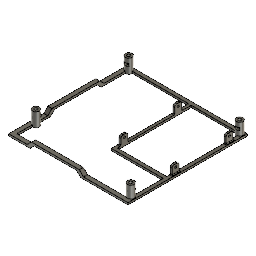
Mobo+HDD (Autodesk Fusion 360 design; units mm, degrees)
Autodesk Fusion 360 part; units mm, degrees
note: some values were not read from the file. Set by a fixed rule: which sketch regions a step uses.
sketch "Sketch4" plane through (0, 0, 0) normal (0, 0, 1) x (1, 0, 0)
  line L0 (0, 0) -> (170, 0)
  line L1 (170, 0) -> (170, 170)
  line L2 (170, 170) -> (0, 170)
  line L3 (0, 170) -> (0, 0)
  line L4 (165, 6) -> (165, 165)
  line L5 (165, 165) -> (6, 165)
  line L6 (6, 165) -> (6, 6)
  line L7 (6, 6) -> (165, 6)
  circle A0 centre (6, 33) radius 2.25
  circle A1 centre (6, 33) radius 5
  circle A2 centre (6, 165) radius 2.25
  circle A3 centre (6, 165) radius 5
  circle A4 centre (164, 10) radius 2.25
  circle A5 centre (164, 10) radius 5
  line L8 (165, 165) -> (95, 165)
  line L9 (95, 165) -> (95, 60)
  line L10 (95, 60) -> (165, 60)
  line L11 (165, 60) -> (165, 165)
  line L12 (91, 165) -> (91, 55)
  line L13 (91, 55) -> (165, 55)
  line L14 (0, 50) -> (6, 50)
  line L15 (0, 60) -> (6, 60)
  line L16 (0, 120) -> (6, 120)
  line L17 (0, 130) -> (6, 130)
  line L18 (26.6543, 6) -> (26.6543, 0)
  line L19 (36.6543, 6) -> (36.6543, 0)
  line L20 (96.6543, 6) -> (96.6543, 0)
  line L21 (106.6543, 6) -> (106.6543, 0)
  line L22 (92, 75) -> (95, 75)
  line L23 (95, 75) -> (95, 65)
  line L24 (95, 65) -> (92, 65)
  line L25 (92, 65) -> (92, 75)
  line L26 (165, 65) -> (168, 65)
  line L27 (168, 65) -> (168, 75)
  line L28 (168, 75) -> (165, 75)
  line L29 (165, 75) -> (165, 65)
  line L30 (95, 151.5) -> (92, 151.5)
  line L31 (92, 151.5) -> (92, 141.5)
  line L32 (92, 141.5) -> (95, 141.5)
  line L33 (95, 141.5) -> (95, 151.5)
  line L34 (165, 151.5) -> (168, 151.5)
  line L35 (168, 151.5) -> (168, 141.5)
  line L36 (168, 141.5) -> (165, 141.5)
  line L37 (165, 141.5) -> (165, 151.5)
  circle A6 centre (164, 165) radius 2.25
  circle A7 centre (164, 165) radius 5
  line L38 (6, 165) -> (6, 170) construction
  line L39 (6, 167.5) -> (170, 167.5) construction
  line L40 (165, 165) -> (170, 165) construction
  line L41 (167.5, 165) -> (167.5, 0) construction
  line L42 (6, 6) -> (0, 6) construction
  line L43 (3, 6) -> (3, 170) construction
  circle A8 centre (147, 167.5) radius 1.75
  circle A9 centre (157, 167.5) radius 1.75
  line L44 (147, 169.25) -> (157, 169.25)
  line L45 (157, 165.75) -> (147, 165.75)
  line L46 (0, 85) -> (170, 85) construction
  circle A10 centre (10.9777, 3) radius 1.75
  line L47 (10.9777, 4.75) -> (20.9777, 4.75)
  circle A11 centre (20.9777, 3) radius 1.75
  line L48 (10.9777, 1.25) -> (20.9777, 1.25)
  circle A12 centre (147, 2.5) radius 1.75
  circle A13 centre (157, 2.5) radius 1.75
  line L49 (147, 0.75) -> (157, 0.75)
  line L50 (157, 4.25) -> (147, 4.25)
  line L51 (0, 0) -> (39.1523, 39.1523) construction
  line L52 (0, 0) -> (55.3697, 0) construction
  line L53 (4.75, 10.9777) -> (4.75, 20.9777)
  circle A14 centre (3, 10.9777) radius 1.75
  line L54 (1.25, 10.9777) -> (1.25, 20.9777)
  circle A15 centre (3, 20.9777) radius 1.75
  line L55 (167.5, 12.0207) -> (164, 14.0415)
  line L56 (164, 14.0415) -> (160.5, 12.0207)
  line L57 (160.5, 12.0207) -> (160.5, 7.9793)
  line L58 (160.5, 7.9793) -> (164, 5.9585)
  line L59 (164, 5.9585) -> (167.5, 7.9793)
  line L60 (167.5, 7.9793) -> (167.5, 12.0207)
  line L61 (9.5, 35.0207) -> (6, 37.0415)
  line L62 (6, 37.0415) -> (2.5, 35.0207)
  line L63 (2.5, 35.0207) -> (2.5, 30.9793)
  line L64 (2.5, 30.9793) -> (6, 28.9585)
  line L65 (6, 28.9585) -> (9.5, 30.9793)
  line L66 (9.5, 30.9793) -> (9.5, 35.0207)
  line L67 (9.5, 167.0207) -> (6, 169.0415)
  line L68 (6, 169.0415) -> (2.5, 167.0207)
  line L69 (2.5, 167.0207) -> (2.5, 162.9793)
  line L70 (2.5, 162.9793) -> (6, 160.9585)
  line L71 (6, 160.9585) -> (9.5, 162.9793)
  line L72 (9.5, 162.9793) -> (9.5, 167.0207)
  line L73 (167.5, 167.0207) -> (164, 169.0415)
  line L74 (164, 169.0415) -> (160.5, 167.0207)
  line L75 (160.5, 167.0207) -> (160.5, 162.9793)
  line L76 (160.5, 162.9793) -> (164, 160.9585)
  line L77 (164, 160.9585) -> (167.5, 162.9793)
  line L78 (167.5, 162.9793) -> (167.5, 167.0207)
  line L79 (160.5, 162.9793) -> (160.5, 161.4293)
  line L80 (167.5, 162.9793) -> (167.5, 161.4293)
  line L81 (167.5, 12.0207) -> (167.5, 13.5707)
  line L82 (160.5, 12.0207) -> (160.5, 13.5707)
  line L83 (9.5, 35.0207) -> (9.5, 36.5707)
  line L84 (2.5, 35.0207) -> (2.5, 36.5707)
  line L85 (2.5, 162.9793) -> (2.5, 161.4293)
  line L86 (9.5, 162.9793) -> (9.5, 161.4293)
  line L87 (1.25, 145.7335) -> (1.25, 155.7335)
  circle A16 centre (3, 155.7335) radius 1.75
  line L88 (4.75, 145.7335) -> (4.75, 155.7335)
  circle A17 centre (3, 145.7335) radius 1.75
  point P0 (6, 33)
  point P1 (164, 10)
  point P2 (164, 165)
  point P3 (164, 10)
  point P4 (6, 33)
  point P5 (6, 165)
  point P6 (164, 165)
  dimension "d44" = 170
  dimension "d45" = 170
  dimension "d47" = 33
  dimension "d48" = 10
  dimension "d49" = 4.5
  dimension "d50" = 10
  dimension "d51" = 4.5
  dimension "d52" = 10
  dimension "d55" = 4.5
  dimension "d56" = 10
  dimension "d57" = 70
  dimension "d58" = 105
  dimension "d60" = 60
  dimension "d61" = 10
  dimension "d63" = 10
  dimension "d64" = 10
  dimension "d65" = 10
  dimension "d66" = 60
  dimension "d67" = 105
  dimension "d75" = 5
  dimension "d76" = 6
  dimension "d77" = 6
  dimension "d78" = 5
  dimension "d79" = 6
  dimension "d80" = 4
  dimension "d81" = 3
  dimension "d82" = 10
  dimension "d83" = 10
  dimension "d84" = 3
  dimension "d85" = 10
  dimension "d86" = 3
  dimension "d87" = 3
  dimension "d88" = 10
  dimension "d89" = 13.5
  dimension "d90" = 13.5
  dimension "d91" = 66.5
  dimension "d92" = 66.5
  dimension "d93" = 6
  dimension "d94" = 4.5
  dimension "d95" = 10
  dimension "d112" = 3.5
  dimension "d113" = 3.5
  dimension "d114" = 10
  dimension "d115" = 8
  dimension "d116" = 45
  dimension "d117" = 10
  dimension "d118" = 3.5
  dimension "d119" = 3.5
  dimension "d121" = 3.5
  dimension "d122" = 3.5
  dimension "d123" = 3.5
  dimension "d124" = 3.5
  dimension "d133" = 10
  dimension "d134" = 3.5
  dimension "d135" = 3.5
  constraint horizontal L0
  constraint vertical L1
  constraint horizontal L2
  constraint vertical L3
  constraint coincident L0.start L3.end
  constraint coincident L6 P4
  constraint coincident P4 P0
  constraint coincident P5 L5.end
  constraint concentric A2 A3
  constraint coincident P3 P1
  constraint horizontal L8
  constraint vertical L9
  constraint horizontal L10
  constraint vertical L11
  constraint parallel L9 L12
  constraint parallel L10 L13
  constraint coincident L5 L12.start
  constraint coincident L4 L13.end
  constraint coincident L3 L14.start
  constraint coincident L6 L14.end
  constraint perpendicular L6 L14
  constraint coincident L3 L15.start
  constraint coincident L6 L15.end
  constraint perpendicular L6 L15
  constraint coincident L3 L16.start
  constraint coincident L6 L16.end
  constraint perpendicular L6 L16
  constraint coincident L3 L17.start
  constraint coincident L6 L17.end
  constraint perpendicular L6 L17
  constraint coincident L7 L18.start
  constraint coincident L0 L18.end
  constraint perpendicular L0 L18
  constraint coincident L7 L19.start
  constraint coincident L0 L19.end
  constraint perpendicular L0 L19
  constraint coincident L7 L21.start
  constraint coincident L0 L21.end
  constraint perpendicular L0 L21
  constraint coincident L0 L20.end
  constraint coincident L7 L20.start
  constraint parallel L1 L4
  constraint parallel L2 L5
  constraint parallel L3 L6
  constraint parallel L0 L7
  constraint horizontal L22
  constraint vertical L23
  constraint horizontal L24
  constraint vertical L25
  constraint coincident L9 L23.end
  constraint horizontal L26
  constraint vertical L27
  constraint horizontal L28
  constraint vertical L29
  constraint coincident L4 L26.start
  constraint horizontal L30
  constraint vertical L31
  constraint horizontal L32
  constraint vertical L33
  constraint coincident L9 L30.start
  constraint horizontal L34
  constraint vertical L35
  constraint horizontal L36
  constraint vertical L37
  constraint coincident L11 L34.start
  constraint coincident L5 P6
  constraint coincident L8 P6
  constraint coincident P6 P2
  constraint coincident L2 L38.end
  constraint coincident A3 L38.end
  constraint perpendicular L2 L38
  constraint midpoint L38 L39.start
  constraint coincident L1 L39.end
  constraint perpendicular L1 L39
  constraint coincident L1 L40.end
  constraint perpendicular L1 L40
  constraint midpoint L40 L41.start
  constraint coincident L0 L41.end
  constraint perpendicular L0 L41
  constraint coincident L3 L42.end
  constraint perpendicular L3 L42
  constraint midpoint L42 L43.start
  constraint coincident L2 L43.end
  constraint perpendicular L2 L43
  constraint coincident L39 A8.centre
  constraint coincident L39 A9.centre
  constraint coincident A8 L44.start
  constraint coincident A9 L44.end
  constraint tangent A9 L44
  constraint parallel L2 L44
  constraint coincident A9 L45.start
  constraint coincident A8 L45.end
  constraint tangent A8 L45
  constraint parallel L2 L45
  constraint midpoint L3 L46.start
  constraint midpoint L1 L46.end
  constraint symmetric A8 L46 A12
  constraint symmetric A9 L46 A13
  constraint symmetric L44.start L46 L49.start
  constraint symmetric L44.end L46 L49.end
  constraint symmetric L45.start L46 L50.start
  constraint symmetric L45.end L46 L50.end
  constraint horizontal L52
  constraint symmetric A10 L51 A14
  constraint symmetric L47.start L51 L53.start
  constraint symmetric L47.end L51 L53.end
  constraint symmetric A11 L51 A15
  constraint symmetric L48.start L51 L54.start
  constraint symmetric L48.end L51 L54.end
  constraint coincident L43 A14.centre
  constraint coincident L43 A15.centre
  constraint coincident L53.end A15
  constraint tangent L53 A15
  constraint coincident L53.start A14
  constraint tangent L53 A14
  constraint coincident A14 L54.start
  constraint tangent A14 L54
  constraint coincident L54.end A15
  constraint tangent L54 A15
  constraint coincident A7 L79.end
  constraint parallel L75 L79
  constraint coincident A7 L80.end
  constraint coincident L41 L80.end
  constraint parallel L41 L80
  constraint coincident L41 L81.end
  constraint coincident A5 L81.end
  constraint parallel L41 L81
  constraint coincident A5 L82.end
  constraint parallel L57 L82
  constraint coincident A1 L83.end
  constraint parallel L66 L83
  constraint coincident A1 L84.end
  constraint parallel L63 L84
  constraint coincident A3 L85.end
  constraint parallel L43 L85
  constraint coincident A3 L86.end
  constraint parallel L72 L86
  constraint coincident L88.end A16
  constraint tangent A16 L88
  constraint coincident L88.start A17
  constraint tangent L88 A17
  constraint coincident L87.start A17
  constraint tangent L87 A17
  constraint coincident L87.end A16
  constraint tangent L87 A16
  constraint coincident L43 A16.centre
  constraint coincident L43 A17.centre
  measures "d44" distance of L0.start L2.end
  measures "d45" distance of L0.start L0.end
  measures "d47" distance of L0 P4
  measures "d48" distance of L0 P3
  measures "d49" diameter of A0
  measures "d50" diameter of A1
  measures "d51" diameter of A2
  measures "d52" diameter of A3
  measures "d55" diameter of A4
  measures "d56" diameter of A5
  measures "d57" distance of L4.end L8.end
  measures "d58" distance of L4.end L10.end
  measures "d60" distance of L15 L16
  measures "d61" distance of L16 L17
  measures "d63" distance of L14 L15
  measures "d64" distance of L18 L19
  measures "d65" distance of L20 L21
  measures "d66" distance of L19 L20
  measures "d67" distance of P5 L15
  measures "d75" distance of L2 L5
  measures "d76" distance of L3 L6
  measures "d77" distance of L0 L7
  measures "d78" distance of L1 L4
  measures "d79" distance of L1 P3
  measures "d80" distance of L9 L12
  measures "d81" distance of L22.start L22.end
  measures "d82" distance of L22.start L24.end
  measures "d83" distance of L26.start L28.end
  measures "d84" distance of L26.start L26.end
  measures "d85" distance of L30.start L32.end
  measures "d86" distance of L30.start L30.end
  measures "d87" distance of L34.start L34.end
  measures "d88" distance of L34.start L36.end
  measures "d89" distance of L5 L30
  measures "d90" distance of L8 L34
  measures "d91" distance of L22.start L31.end
  measures "d92" distance of L27.end L35.end
  measures "d93" distance of L1 P6
  measures "d94" diameter of A6
  measures "d95" diameter of A7
  measures "d112" diameter of A8
  measures "d113" diameter of A9
  measures "d114" distance of A8.centre A9.centre
  measures "d115" horizontal distance of L4.end A9.centre
  measures "d116" angle of L51 L52
  measures "d117" vertical distance of L54.start A15.centre
  measures "d118" diameter of A15
  measures "d119" diameter of A14
  measures "d121" distance of P3 L60
  measures "d122" distance of P4 L66
  measures "d123" distance of P5 L72
  measures "d124" distance of P6 L78
  measures "d133" vertical distance of A16.centre L87.start
  measures "d134" diameter of A16
  measures "d135" diameter of A17
extrude "Extrude8" add sketch "Sketch4" along normal blind 3 contours L0 L3 L6 L7 A1 L14 L18 | L0 L7 L18 L19 | L3 L6 L14 L15 | L0 L7 L20 L21 | L3 L6 L16 L17 | L6 A1 L61 L83 | L6 A1 L62 L84 | L0 L1 L2 L4 L7 A5 L11 L21 L26 L27 L28 L34 L35 L36 A7 | L6 A1 L63 L64 L84 | L6 A1 L65 L66 L83 | L2 L3 L6 A3 L17 | L6 A0 L61 L65 L66 | L6 A0 L62 L63 L64 | L6 A0 | L6 A0 | L7 A5 L57 L58 L82 | L4 L7 A5 L58 L59 L60 L81 | L2 L5 A3 L8 A7 | L5 A3 L67 L68 L69 L72 L85 | L6 A3 L70 L85 | L6 A3 L71 L86 | L5 L8 A7 L73 L74 L75 L78 L80 | L4 L7 A4 L55 L56 L57 L58 L59 | L7 L58 L59 | L4 A5 L55 L56 L82 | L5 A3 L72 L86 | L5 L6 A2 L67 L68 L69 L70 L72 | L5 L6 A2 L71 L72 | L5 L8 A7 L75 L79 | L4 L7 L59 | L4 A5 L55 L81 | L4 L5 L9 L10 L12 L13 L22 L24 L25 L30 L31 L32 | L5 L6 A2 | L5 L6 A2 | L4 L11 A7 L77 L80 | L4 L5 L8 L11 A6 L73 L74 L75 L77 L78 | L4 L5 L8 L11 A6 L75 L76 L77 | L4 L11 A7 L76 L77 L79 | L4 A4 L55 L59 L60 | L4 L5 L8 L11 A6 | L4 L5 L8 L11 A6 | L9 L30 L31 L32 L33 | L4 A4 | L4 A4 | L4 L11 L34 L35 L36 L37 | L4 L11 L26 L27 L28 L29 | L9 L22 L23 L24 L25 | A8 | A8 A9 L44 L45 | A9 | A10 | A10 L47 A11 L48 | A11 | A12 | A12 A13 L49 L50 | A13 | L53 A14 L54 A15 | A14 | A15 | L87 A16 L88 A17 | A17 | A16 makes body 1 at (2, 29.3333, 0) makes body 2 at (142.5514, 2, 0)
extrude "Extrude9" add sketch "Sketch4" along normal blind 20 contours L6 A1 L61 L83 | L6 A1 L62 L84 | L6 A1 L63 L64 L84 | L6 A1 L65 L66 L83 | L6 A0 L61 L65 L66 | L6 A0 L62 L63 L64 | L7 A5 L57 L58 L82 | L4 L7 A5 L58 L59 L60 L81 | L5 A3 L67 L68 L69 L72 L85 | L6 A3 L70 L85 | L6 A3 L71 L86 | L5 L8 A7 L73 L74 L75 L78 L80 | L4 L7 A4 L55 L56 L57 L58 L59 | L7 L58 L59 | L4 A5 L55 L56 L82 | L5 A3 L72 L86 | L5 L6 A2 L67 L68 L69 L70 L72 | L5 L6 A2 L71 L72 | L5 L8 A7 L75 L79 | L4 L7 L59 | L4 A5 L55 L81 | L4 L11 A7 L77 L80 | L4 L5 L8 L11 A6 L73 L74 L75 L77 L78 | L4 L5 L8 L11 A6 L75 L76 L77 | L4 L11 A7 L76 L77 L79 | L4 A4 L55 L59 L60 bodies 2 1
extrude "Extrude14" add sketch "Sketch4" along normal blind 7 contours L0 L7 L18 L19 | L3 L6 L14 L15 | L0 L7 L20 L21 | L3 L6 L16 L17 bodies 2 1
extrude "Extrude10" add sketch "Sketch4" along normal blind 3 from surface at 6 contours L0 L7 L18 L19 | L3 L6 L14 L15 | L0 L7 L19 L20 | L3 L6 L15 L16 | L0 L7 L20 L21 | L3 L6 L16 L17 bodies 2 1
extrude "Extrude11" add sketch "Sketch4" along normal blind 15 contours L9 L30 L31 L32 L33 | L4 L11 L34 L35 L36 L37 | L4 L11 L26 L27 L28 L29 | L9 L22 L23 L24 L25 bodies 2
sketch "Sketch5" plane through (168, 0, 0) normal (1, 0, 0) x (0, 1, 0)
  line L0 (141.5, 3) -> (151.5, 3)
  line L1 (151.5, 3) -> (151.5, 15)
  line L2 (151.5, 15) -> (141.5, 15)
  line L3 (141.5, 15) -> (141.5, 3)
  circle A0 centre (146.5, 11) radius 1.5
  line L4 (65, 3) -> (75, 3)
  line L5 (75, 3) -> (75, 15)
  line L6 (75, 15) -> (65, 15)
  line L7 (65, 15) -> (65, 3)
  circle A1 centre (70, 11) radius 1.5
  dimension "d98" = 3
  dimension "d99" = 4
  dimension "d100" = 5
  dimension "d101" = 3
  dimension "d102" = 4
  dimension "d120" = 76.5
  measures "d98" diameter of A0
  measures "d99" distance of L2 A0.centre
  measures "d100" distance of L1 A0.centre
  measures "d101" diameter of A1
  measures "d102" distance of L6 A1.centre
  measures "d120" distance of A0.centre A1.centre
extrude "Extrude12" cut sketch "Sketch5" against normal blind 80 contours A0 | A1 bodies 2
extrude "Extrude13" cut sketch "Sketch4" along normal blind 3.5 from surface at 10 contours L6 A1 L61 L83 | L6 A1 L62 L84 | L6 A0 L61 L65 L66 | L6 A0 L62 L63 L64 | L6 A3 L70 L85 | L6 A3 L71 L86 | L4 L7 A4 L55 L56 L57 L58 L59 | L4 A5 L55 L56 L82 | L5 L6 A2 L67 L68 L69 L70 L72 | L5 L6 A2 L71 L72 | L4 A5 L55 L81 | L4 L11 A7 L77 L80 | L4 L5 L8 L11 A6 L73 L74 L75 L77 L78 | L4 L5 L8 L11 A6 L75 L76 L77 | L4 L11 A7 L76 L77 L79 | L4 A4 L55 L59 L60 bodies 2
chamfer "Chamfer2" distance 6 angle 45 8 edges at (3, 130, 9) (3, 50, 9) (26.6543, 3, 9) (106.6543, 3, 9) (3, 120, 0) (3, 60, 0) (36.6543, 3, 0) (96.6543, 3, 0) on bodies 2
fillet "Fillet1" radius 1 12 edges at (93.5, 75, 3) (93.5, 65, 3) (92, 70, 3) (93.5, 141.5, 3) (93.5, 151.5, 3) (92, 146.5, 3) (166.5, 151.5, 3) (168, 146.5, 3) (166.5, 141.5, 3) (166.5, 75, 3) (168, 70, 3) (166.5, 65, 3) on bodies 2
fillet "Fillet1" radius 3 8 edges at (93.5, 65, 15) (93.5, 75, 15) (93.5, 141.5, 15) (93.5, 151.5, 15) (166.5, 151.5, 15) (166.5, 141.5, 15) (166.5, 75, 15) (166.5, 65, 15) on bodies 2
named bodies: "Mini-ITX"
